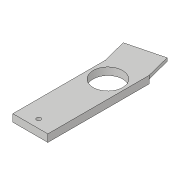
# Autodesk Inventor part: Lidar Sensor CAse Piece 1
Saved by Autodesk Inventor 2018.3 (Build 223284000, 284)
## iProperties
Created: 2019-02-15
Part Number: Lidar Sensor CAse Piece 1
Material: Generic
Document SubType Name: Modeling
Designer: aye06091
Mass: 11.1601 g
Surface Area: 60.4599 cm^2
Volume: 11.1601 cm^3
Density: 1 g/cm^3
Appearance: Default
Author: aye06091
Autodesk Inventor part; units mm, degrees
ref_plane "YZ Plane" through (0, 0, 0) normal (1, 0, 0) x (0, 1, 0)
ref_plane "XZ Plane" through (0, 0, 0) normal (0, 1, 0) x (-1, 0, 0)
ref_plane "XY Plane" through (0, 0, 0) normal (0, 0, 1) x (1, 0, 0)
sketch "Sketch1" plane through (0, 0, 0) normal (0, 1, 0) x (-1, 0, 0)
  line L0 (18.6455, 5.0782) -> (18.6456, 5.0782)
  line L1 (-29.4725, -45.6897) -> (-2.9825, -38.9263)
  circle A0 centre (-20.9401, -9.3559) radius 11.176
  line L2 (-7.6951, 49.3816) -> (-7.6951, -20.4684)
  line L3 (-7.6951, -20.4684) -> (-2.9825, -38.9263)
  line L4 (-2.9825, -38.9263) -> (-29.4725, -45.6897)
  line L5 (-29.4725, -45.6897) -> (-34.1852, -27.2318)
  line L6 (-34.1852, -27.2318) -> (-34.1852, 49.3816)
  line L7 (-34.1852, 49.3816) -> (-7.6951, 49.3816)
  dimension "d4" = 22.352
  dimension "d30" = 19.05
  dimension "d32" = 19.05
  dimension "d33" = 26.49
  dimension "d35" = 13.245
  dimension "d36" = 58.7375
  dimension "d37" = 69.85
  dimension "d42" = 75.677
  constraints: 16 end point, 3 perpendicular, 2 vertical, 1 centre point, 1 parallel
  measures "d4" diameter of A0
  measures "d30" distance of L2.end L1.end
  measures "d32" distance of L1.start L5.end
  measures "d33" distance of L6.end L2.start
  measures "d35" distance from line of A0.centre L2
  measures "d36" distance from line of L7 A0.centre
  measures "d37" distance of L2.start L2.end
  measures "d42" angle of L6 L1
extrude "Extrusion1" add sketch "Sketch1" along normal blind 5.6134
sketch "Sketch4" plane through (0, 5.6134, 0) normal (0, 1, 0) x (1, 0, 0)
  line L0 (7.6951, -49.3816) -> (34.1852, -49.3816) projected
  circle A0 centre (20.9401, -43.0316) radius 1.6002
  point P0 (0, 0)
  dimension "d38" = 3.2004
  dimension "d39" = 6.35
  constraints: 1 centre point
  measures "d38" diameter of A0
  measures "d39" distance from line of L0 A0.centre
extrude "Extrusion4" cut sketch "Sketch4" against normal blind 25.4
sketch "Sketch5" plane through (0, 0, 0) normal (0, -1, 0) x (1, 0, 0)
  line L0 (29.4725, -45.6897) -> (34.1852, -27.2318) projected
  line L1 (34.1852, -27.2318) -> (7.6951, -20.4684)
  line L2 (7.6951, -20.4684) -> (6.9474, -23.3971)
  line L3 (6.9474, -23.3971) -> (30.718, -29.4662)
  line L4 (33.4374, -30.1605) -> (34.1852, -27.2318)
  line L5 (34.1852, 49.3816) -> (34.1852, -27.2318) projected
  line L6 (34.1852, -27.2318) -> (29.4725, -45.6897)
  line L7 (29.4725, -45.6897) -> (26.753, -44.9954)
  line L8 (26.753, -44.9954) -> (30.718, -29.4662)
  line L9 (7.6951, -20.4684) -> (34.1852, -27.2318)
  point P0 (0, 0)
  dimension "d46" = 3.0226
  dimension "d47" = 2.8067
  constraints: 16 end point, 4 parallel, 2 perpendicular, 1 collinear, 1 point on line
  measures "d46" distance between parallel lines of L1 L3
  measures "d47" distance between parallel lines of L8 L0
extrude "Extrusion5" cut sketch "Sketch5" against normal blind 3.175
body "Solid1"
